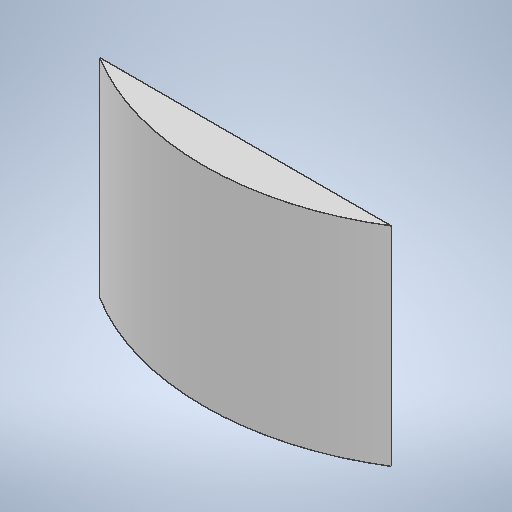
# Autodesk Inventor part: ball
Saved by Autodesk Inventor 2025 (Build 290162000, 162)
## iProperties
Created: 2025-10-18
Part Number: ball
Material: 一般
Document SubType Name: Modeling
Designer: sooo1
Density: 1 g/cm^3
Appearance: 既定
Author: sooo1
Autodesk Inventor part; units mm, degrees
ref_plane "YZ Plane" through (0, 0, 0) normal (1, 0, 0) x (0, 1, 0)
ref_plane "XZ Plane" through (0, 0, 0) normal (0, 1, 0) x (-1, 0, 0)
ref_plane "XY Plane" through (0, 0, 0) normal (0, 0, 1) x (1, 0, 0)
sketch "スケッチ1" plane through (0, 0, 0) normal (0, 1, 0) x (-1, 0, 0)
  circle A0 centre (0, 0) radius 6.625
  line L0 (9.275, 0) -> (-9.275, 0) projected
  line L1 (3.5, 5.625) -> (-3.5, 5.625)
  line L2 (5.3064, 6.625) -> (-3.654, 6.625)
  dimension "d0" = 1
  dimension "d1" = 7
  constraints: 4 end point, 2 parallel, 2 point on circle, 1 centre point, 1 coincident, 1 tangent
  measures "d0" distance between parallel lines of L2 L1
  measures "d1" distance of L1.start L1.end
extrude "押し出し1" add sketch "スケッチ1" along normal mid plane 5 contours L1 A0
sketch "スケッチ2" plane through (3.5, -2.5, 5.625) normal (0, 0, -1) x (-1, 0, 0)
  line L0 (7, 0) -> (0, 0) projected
  line L1 (7, 5) -> (7, 0) projected
  line L2 (0, 5) -> (7, 5) projected
  line L3 (0, 0) -> (0, 5) projected
  line L4 (4.95, 5) -> (4.95, 0)
  line L5 (2.05, 5) -> (2.05, 0)
  line L6 (3.5, 2.5) -> (3.5, 5)
  line L7 (4.95, 3.1) -> (2.05, 3.1)
  line L8 (4.95, 1.9) -> (2.05, 1.9)
  dimension "d4" = 2.9
  dimension "d5" = 1.45
  dimension "d8" = 1.9
  dimension "d9" = 1.2
  constraints: 10 end point, 8 point on line, 4 perpendicular, 1 midpoint
  measures "d4" distance between parallel lines of L5 L4
  measures "d5" distance between parallel lines of L6 L4
  measures "d8" distance between parallel lines of L2 L7
  measures "d9" distance between parallel lines of L8 L7
extrude "押し出し2" add sketch "スケッチ2" along normal blind 1.5 contours L8 L5 L7 L4
